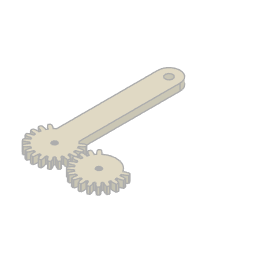
Workshop File v2 (Autodesk Fusion 360 design; units mm, degrees)
Autodesk Fusion 360 part; units mm, degrees
sketch "Sketch1" plane through (0, 0, 0) normal (0, 1, 0) x (1, 0, 0)
  circle A0 centre (0, 0) radius 1.95 construction
  line L0 (0, 0) -> (0, 0.05)
  circle A1 centre (0, 0) radius 12.5
  line L1 (0, 0) -> (0, 12.5) construction
  line L2 (0.3327, 1.565) -> (2.5989, 12.2268)
  line L3 (0, 1.95) -> (0.3327, 1.565)
  line L4 (0, 1.95) -> (-0.3327, 1.565)
  line L5 (-0.3327, 1.565) -> (-2.5989, 12.2268)
  arc A2 (-0.3327, 1.565) -> (0.3327, 1.565) centre (0, 0) ccw construction
  line L6 (0, 0) -> (12.5, 0) construction
  dimension "d1" = 3.9
  dimension "d2" = 3.2
  dimension "d3" = 10.55
  dimension "d4" = 12
  constraint coincident A0.centre L0.start
  constraint concentric A0 A2
  constraint vertical L0
  constraint coincident A1 L1.end
  constraint parallel L0 L1
  constraint coincident A1 L2.end
  constraint coincident A0 L3.start
  constraint coincident L1 L3.start
  constraint symmetric L1 L2.end L5.end
  constraint symmetric L1 L3.start L4.start
  constraint symmetric L1 L2.start L4.end
  constraint coincident A1 L6.end
  constraint perpendicular L0 L6
  measures "d1" diameter of A0
  measures "d2" diameter of A2
  measures "d4" angle of L1 L2
extrude "Extrude1" add sketch "Sketch1" along normal blind 5 contours A1 L2 L3 L4 L5 picked at (0, 8.963) makes body 1
pattern_circular "C-Pattern1" count 15 over 360 about axis through (0, 1.75, 0) along (0, 1, 0) of bodies 1 makes body 2 at (-1.0881, 1.6667, -5.119) makes body 3 at (-6.6608, 0, -5.9974) makes body 4 at (-8.5244, 0, -2.7697) makes body 5 at (-8.9139, 0, 0.9369) makes body 6 at (-7.7622, 0, 4.4815) makes body 7 at (-5.2683, 0, 7.2512) makes body 8 at (-1.8635, 0, 8.7672) makes body 9 at (1.8635, 0, 8.7672) makes body 10 at (5.2683, 0, 7.2512) makes body 11 at (7.7622, 0, 4.4815) makes body 12 at (8.9139, 0, 0.9369) makes body 13 at (8.5244, 0, -2.7697) makes body 14 at (6.6608, 0, -5.9974) makes body 15 at (1.0881, 1.6667, -5.119)
combine "Combine1" operation add target body 1 tool bodies 11 12 2 6 15 4 13 5 7 14 10 8 3 9
fillet "Fillet2" radius 0.1 29 edges at (-0.3327, 2.5, -1.565) (0, 2.5, -1.95) (0.3327, 2.5, -1.565) (0.7931, 2.5, -1.7814) (0.9405, 2.5, -1.2944) (1.4491, 2.5, -1.3048) (1.3856, 2.5, -0.8) (1.8546, 2.5, -0.6026) (1.5912, 2.5, -0.1672) (1.9393, 2.5, 0.2038) (1.5217, 2.5, 0.4944) (1.189, 2.5, 1.0706) (1.1462, 2.5, 1.5776) (0.6508, 2.5, 1.4617) (0.4054, 2.5, 1.9074) (0, 2.5, 1.6) (-0.4054, 2.5, 1.9074) (-0.6508, 2.5, 1.4617) (-1.1462, 2.5, 1.5776) (-1.189, 2.5, 1.0706) (-1.6887, 2.5, 0.975) (-1.5217, 2.5, 0.4944) (-1.9393, 2.5, 0.2038) (-1.5912, 2.5, -0.1672) (-1.8546, 2.5, -0.6026) (-1.3856, 2.5, -0.8) (-1.4491, 2.5, -1.3048) (-0.9405, 2.5, -1.2944) (-0.7931, 2.5, -1.7814) on bodies 1
fillet "Fillet2" radius 0.1 1 edges at (1.6887, 2.5, 0.975) on bodies 1
sketch "Sketch2" plane through (0, 0, 0) normal (0, 1, 0) x (1, 0, 0)
  circle A0 centre (0, 0) radius 1.6
  circle A1 centre (0, 0) radius 1.95
  line L0 (8, 0) -> (8, 82.5)
  arc A2 (8, 82.5) -> (-8, 82.5) centre (0, 82.5) ccw
  line L1 (-8, 82.5) -> (-8, 0)
  arc A3 (-8, 0) -> (8, 0) centre (0, 0) ccw
  line L2 (0, 0) -> (0, 82.5) construction
  circle A4 centre (0, 82.5) radius 2.75
  line L3 (0, 0) -> (16.5, 0)
  line L4 (0, 0) -> (14.3215, -2.2683) construction
  line L5 (0, 0) -> (16.4774, -0.8635) construction
  line L6 (0, 0) -> (1.5978, -0.0837)
  line L7 (0, 0) -> (12.4315, -1.3066) construction
  line L8 (16.5, 0) -> (12.5, 0)
  circle A5 centre (0, 0) radius 12.5 construction
  arc A6 (12.6251, -1.325) -> (16.345, -0.9068) centre (13.4341, 8.2323) ccw
  arc A7 (16.345, -0.9068) -> (16.4841, -0.725) centre (16.2843, -0.7162) ccw
  arc A8 (12.4829, -0.6542) -> (12.4096, -1.5003) centre (0, 0) ccw
  arc A9 (12.6251, -1.325) -> (12.4096, -1.5003) centre (12.6082, -1.5243) ccw
  arc A10 (16.4841, -0.725) -> (16.5, 0) centre (0, 0) ccw
  arc A11 (8, 14.4309) -> (-8, 14.4309) centre (0, 0) ccw
  arc A12 (8, 12.0934) -> (-8, 12.0934) centre (0, 0) ccw construction
  circle A13 centre (0, 0) radius 12.5
  arc A14 (16.345, 0.9068) -> (12.6251, 1.325) centre (13.4341, -8.2323) ccw
  arc A15 (12.4096, 1.5003) -> (12.6251, 1.325) centre (12.6082, 1.5243) ccw
  arc A16 (16.5, 0) -> (16.4841, 0.725) centre (0, 0) ccw
  arc A17 (16.4841, 0.725) -> (16.345, 0.9068) centre (16.2843, 0.7162) ccw
  dimension "d15" = 25
  dimension "d16" = 3.2
  dimension "d17" = 3.9
  dimension "d18" = 5.5
  dimension "d19" = 8
  dimension "d24" = 3
  dimension "d25" = 6
  dimension "d26" = 9
  dimension "d27" = 4
  dimension "d29" = 0.2
  dimension "d30" = 0.2
  constraint coincident A0.centre A1.centre
  constraint concentric A0 A8
  constraint tangent L0 A2
  constraint tangent A2 L1
  constraint parallel L0 L1
  constraint tangent L1 A3
  constraint tangent L0 A3
  constraint vertical L2
  constraint concentric A2 A4
  constraint coincident L5 L6.end
  constraint coincident A0 L6.end
  constraint horizontal L3
  constraint coincident L3 L8.end
  constraint coincident L8.end A8
  constraint tangent L7 A6
  constraint coincident L5.end A10
  constraint coincident L5.end A6
  constraint tangent A7 A10
  constraint tangent A6 A7
  constraint coincident L5 A8.start
  constraint coincident L7.end A6
  constraint coincident L7.end A8
  constraint tangent A6 A9
  constraint tangent A8 A9
  constraint coincident L0 A11.start
  constraint concentric A10 A11
  constraint coincident L1 A11.end
  constraint coincident L1 A12.end
  constraint coincident L0 A12.start
  constraint concentric A1 A13
  constraint coincident L8.end A13
  constraint symmetric L8.start L3 A10.end
  constraint symmetric L3 A6 A14
  constraint symmetric L3 A7.end A16.end
  constraint symmetric L3 A6.end A14.start
  constraint symmetric L3 A7 A17
  constraint symmetric L3 A6.start A14.end
  constraint symmetric L3 A8.end A15.start
  constraint symmetric L3 A9 A15
  constraint symmetric L3 A10 A16
  measures "d15" diameter of A8
  measures "d16" diameter of A0
  measures "d17" diameter of A1
  measures "d18" diameter of A4
  measures "d19" distance of L0 L2
  measures "d24" angle of L3 L5
  measures "d25" angle of L3 L7
  measures "d26" angle of L3 L4
  measures "d27" distance of L3.end L8.end
  measures "d29" radius of A7
  measures "d30" radius of A9
extrude "Extrude3" add sketch "Sketch2" along normal blind 5 separate body contours L3 L8 A8 A13 A14 A15 A16 A17 | L3 L8 A6 A7 A8 A9 A10 A13 makes body 16
pattern_circular "C-Pattern2" count 20 over 360 about axis through (0, 1.75, 0) along (0, 1, 0) of bodies 16 makes body 17 at (13.1896, 3.3333, -5.6737) makes body 18 at (10.0916, 1.6667, -9.0119) makes body 19 at (7.618, 1.6667, -12.6519) makes body 20 at (3.9519, 1.6667, -15.4799) makes body 21 at (-1.3202, 3.3333, -14.2974) makes body 22 at (-5.6737, 3.3333, -13.1896) makes body 23 at (-8.7595, 3.3333, -9.7577) makes body 24 at (-12.3428, 3.3333, -7.3357) makes body 25 at (-15.4799, 1.6667, -3.9519) makes body 26 at (-14.2974, 3.3333, 1.3202) makes body 27 at (-11.9869, 3.3333, 5.3155) makes body 28 at (-10.7908, 3.3333, 9.4719) makes body 29 at (-6.5733, 3.3333, 11.3461) makes body 30 at (-3.9519, 1.6667, 15.4799) makes body 31 at (1.3202, 3.3333, 14.2974) makes body 32 at (5.3155, 3.3333, 11.9869) makes body 33 at (9.4719, 3.3333, 10.7908) makes body 34 at (12.3428, 3.3333, 7.3357) makes body 35 at (14.0056, 3.3333, 3.1625)
combine "Combine3" operation add target body 1 tool bodies 18 17 16 35 34 33 32 31 30 29 28 27 26 25 24
ref_plane "WorkPlane1" through (16, 0, 0) normal (1, 0, 0) x (0, 1, 0)
mirror "Mirror1" about plane through (16, 0, 0) normal (1, 0, 0) of bodies 1 makes body 36
extrude "Extrude2" add sketch "Sketch2" along normal blind 5 contours L0 A2 L1 A11 | L0 L1 A8 A11 A13 bodies 1
move_body "Move1" bodies 36 to x (0.984808, 0, 0.173648) y (0, 1, 0) z (-0.173648, 0, 0.984808) at (0.4862, 0, -5.5567)
fillet "Fillet3" [rolled back] radius 5
hidden bodies 19 20 21 22 23
equation "d3 = 5.05 mm + 5.5 mm"
